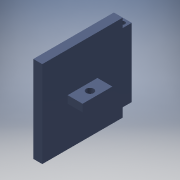
# Autodesk Inventor part: membre_pince
Saved by Autodesk Inventor 2017 SP1 (Build 210196100, 196)
## iProperties
Part Number: membre_pince
Material: Plastique PC/ABS
Document SubType Name: Modeling
Designer: Biscuit
Density: 0.357273 g/cm^3
Appearance: Caoutchouc - Bleu
Author: Biscuit
Autodesk Inventor part; units mm, degrees
ref_plane "YZ Plane" through (0, 0, 0) normal (1, 0, 0) x (0, 1, 0)
ref_plane "XZ Plane" through (0, 0, 0) normal (0, 1, 0) x (-1, 0, 0)
ref_plane "XY Plane" through (0, 0, 0) normal (0, 0, 1) x (1, 0, 0)
sketch "Esquisse1" plane through (0, 0, 0) normal (1, 0, 0) x (0, 1, 0)
  line L0 (0, 0) -> (58, 0)
  line L1 (58, 0) -> (58, -58)
  line L2 (58, -58) -> (0, -58)
  line L3 (0, -58) -> (0, 0)
  line L4 (50, 0) -> (58, 0)
  line L5 (58, 0) -> (58, -6)
  line L6 (58, -6) -> (50, -6)
  line L7 (50, -6) -> (50, 0)
  line L8 (58, -52) -> (50, -52)
  line L9 (50, -52) -> (50, -58)
  line L10 (50, -58) -> (58, -58)
  line L11 (58, -58) -> (58, -52)
  dimension "d0" = 58
  dimension "d1" = 58
  dimension "d2" = 6
  dimension "d3" = 8
  dimension "d4" = 8
  dimension "d5" = 6
  dimension "d15" = 46
  constraints: 24 end point, 6 parallel, 5 point on line, 3 horizontal, 3 perpendicular
  measures "d0" distance of L0.end L1.end
  measures "d1" distance of L1.end L2.end
  measures "d2" distance of L6.end L4.start
  measures "d3" distance of L5.end L6.end
  measures "d4" distance of L8.start L8.end
  measures "d5" distance of L8.end L9.end
  measures "d15" distance between parallel lines of L6 L8
extrude "Extrusion1" add sketch "Esquisse1" along normal blind 6 contours L0 L7 L6 L1 L8 L9 L2 L3
sketch "Esquisse2" plane through (0, 50, -6) normal (0, 0, 1) x (1, 0, 0)
  circle A0 centre (3, 5) radius 1.5
  line L0 (6, 8) -> (6, 0) projected
  line L1 (0, 8) -> (0, 0) projected
  line L2 (0, 0) -> (6, 0) projected
  line L3 (0, 8) -> (6, 8) projected
  point P0 (0, -50)
  dimension "d8" = 3
  dimension "d9" = 6
  dimension "d10" = 8
  dimension "d11" = 3
  dimension "d32" = 3
  constraints: 1 centre point
  measures "d8" diameter of A0
  measures "d9" distance between parallel lines of L0 L1
  measures "d10" distance between parallel lines of L2 L3
  measures "d11" distance from line of L1 A0.centre
  measures "d32" distance from line of L3 A0.centre
extrude "Extrusion2" cut sketch "Esquisse2" against normal up to next contours A0
sketch "Esquisse3" plane through (6, 0, 0) normal (1, 0, 0) x (0, 0, -1)
  line L0 (21.4, 15) -> (26.4, 15)
  line L1 (26.4, 15) -> (26.4, 35)
  line L2 (26.4, 35) -> (21.4, 35)
  line L3 (21.4, 35) -> (21.4, 15)
  line L4 (0, 50) -> (0, 0) projected
  line L5 (0, 0) -> (58, 0) projected
  line L6 (6, 50) -> (0, 50) projected
  dimension "d16" = 5
  dimension "d17" = 20
  dimension "d18" = 21.4
  dimension "d19" = 15
  dimension "d20" = 50
  dimension "d21" = 58
  constraints: 8 end point, 2 parallel, 1 horizontal, 1 perpendicular
  measures "d16" distance of L0.start L0.end
  measures "d17" distance of L0.end L1.end
  measures "d18" distance between parallel lines of L4 L3
  measures "d19" distance between parallel lines of L5 L0
  measures "d20" distance between parallel lines of L5 L6
  measures "d21" distance of L4.end L5.end
extrude "Extrusion3" add sketch "Esquisse3" along normal blind 10
sketch "Esquisse4" plane through (6, 15, -21.4) normal (0, 0, 1) x (1, 0, 0)
  circle A0 centre (5, 10) radius 2.5
  line L0 (0, 20) -> (10, 20) projected
  line L1 (0, 0) -> (10, 0) projected
  line L2 (10, 20) -> (10, 0) projected
  line L3 (0, 35) -> (0, -15) projected
  point P0 (-6, -15)
  dimension "d24" = 5
  dimension "d25" = 20
  dimension "d26" = 10
  dimension "d27" = 5
  dimension "d28" = 10
  constraints: 1 centre point
  measures "d24" diameter of A0
  measures "d25" distance between parallel lines of L0 L1
  measures "d26" distance between parallel lines of L2 L3
  measures "d27" distance from line of L2 A0.centre
  measures "d28" distance from line of L0 A0.centre
extrude "Extrusion4" cut sketch "Esquisse4" against normal up to next contours A0
fillet "Congé1" radius 3 2 edges at (6, 58, -29) (0, 58, -29)
equation "\"d5\" = d2"
equation "\"d11\" = 0.5 * d9"
equation "\"d19\" = 0.5 * d20 - 0.5 * d17"
equation "\"d27\" = 0.5 * d26"
equation "\"d28\" = 0.5 * d25"
